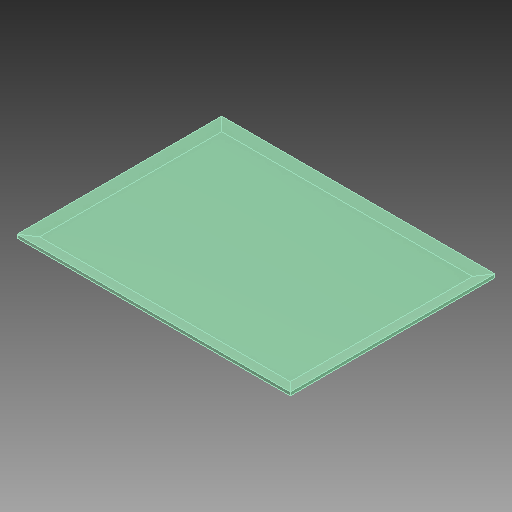
# Autodesk Inventor part: Main
Saved by Autodesk Inventor 2023 (Build 270158000, 158)
## iProperties
Created: 2022-01-17
Part Number: Main
Material: Пластик АБС
Document SubType Name: Modeling
Designer: Администратор
Density: 1.06 g/cm^3
Appearance: Гладкий — темный цвет морской волны
Author: Администратор
Autodesk Inventor part; units mm, degrees
ref_plane "YZ Plane" through (0, 0, 0) normal (1, 0, 0) x (0, 1, 0)
ref_plane "XZ Plane" through (0, 0, 0) normal (0, 1, 0) x (-1, 0, 0)
ref_plane "XY Plane" through (0, 0, 0) normal (0, 0, 1) x (1, 0, 0)
sketch "Эскиз2" plane through (0, 0, 0) normal (0, 1, 0) x (-1, 0, 0)
  line L0 (1215, -910) -> (-1215, -910)
  line L1 (-1215, -910) -> (-1215, 910)
  line L2 (-1215, 910) -> (1215, 910)
  line L3 (1215, 910) -> (1215, -910)
  line L4 (0, -910) -> (0, 910) construction
  line L5 (1215, 0) -> (-1215, 0) construction
  point P0 (0, 0)
  point P1 (0, 0)
  dimension "d14" = 2430
  dimension "d15" = 1820
  constraints: 12 end point, 5 midpoint, 2 parallel, 1 coincident, 1 horizontal, 1 perpendicular
  measures "d14" distance of L0.start L0.end
  measures "d15" distance of L2.end L0.start
extrude "Выдавливание2" add sketch "Эскиз2" against normal blind 10
sketch "Эскиз3" plane through (0, 0, 0) normal (0, 1, 0) x (-1, 0, 0)
  line L0 (-1215, 910) -> (-1215, -910) projected
  line L1 (-1215, -910) -> (1215, -910) projected
  line L2 (1215, -910) -> (1215, 910) projected
  line L3 (1215, 910) -> (-1215, 910) projected
  line L4 (1235, -930) -> (-1235, -930)
  line L5 (-1235, -930) -> (-1235, 930)
  line L6 (-1235, 930) -> (1235, 930)
  line L7 (1235, 930) -> (1235, -930)
  line L8 (1115, -810) -> (-1115, -810)
  line L9 (-1115, -810) -> (-1115, 810)
  line L10 (-1115, 810) -> (1115, 810)
  line L11 (1115, 810) -> (1115, -810)
  dimension "d22" = 20
  dimension "d23" = 100
  constraints: 16 end point, 6 other
  measures "d22" distance between parallel lines of L1 L4
  measures "d23" distance between parallel lines of L1 L8
sketch "Эскиз5" plane through (0, 0, 0) normal (0, 0, 1) x (1, 0, 0)
  line L0 (-1215, 0) -> (-1215, 220) projected
  line L1 (-1215, 0) -> (-1215, 20)
  line L2 (-1215, 20) -> (-1115, 0)
  line L3 (1215, 0) -> (-1215, 0) projected
  line L4 (-1115, 0) -> (-1215, 0)
  point P0 (0, 0)
  dimension "d30" = 20
  constraints: 6 end point, 1 collinear, 1 point on line
  measures "d30" distance of L0.start L1.end
sweep "Сдвиг1" add profiles "Эскиз5" path "Эскиз3" path curves L9 L8 L11 L10
